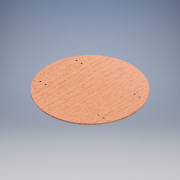
# Autodesk Inventor part: second floor
Saved by Autodesk Inventor 2017 (Build 210142000, 142)
## iProperties
Created: 2019-10-03
Part Number: second floor
Material: Generic
Document SubType Name: Modeling
Designer: User
Density: 1 g/cm^3
Appearance: Weld - Aluminum
Mass: 93.7027 g
Surface Area: 649.465 cm^2
Volume: 93.7027 cm^3
Author: User
Autodesk Inventor part; units mm, degrees
ref_plane "YZ Plane" through (0, 0, 0) normal (1, 0, 0) x (0, 1, 0)
ref_plane "XZ Plane" through (0, 0, 0) normal (0, 1, 0) x (-1, 0, 0)
ref_plane "XY Plane" through (0, 0, 0) normal (0, 0, 1) x (1, 0, 0)
sketch "Sketch1" plane through (0, 0, 0) normal (0, 0, 1) x (1, 0, 0)
  circle A0 centre (0, 0) radius 100
  dimension "d0" = 200
  constraints: 1 centre point, 1 coincident
  measures "d0" diameter of A0
extrude "Extrusion2" add sketch "Sketch1" along normal blind 3
ref_plane "Work Plane1" through (-33, -35, 0) normal (-1, 0, 0) x (0, 0, 1)
sketch "Sketch33" plane through (0, 0, 0) normal (0, 0, -1) x (-1, 0, 0)
  line L0 (-60, 40) -> (-78, 40)
  line L1 (-78, 40) -> (-78, 46)
  line L2 (-78, 46) -> (-60, 46)
  line L3 (-60, 46) -> (-60, 40)
  point P0 (0, 0)
  dimension "d123" = 18
  dimension "d124" = 6
  constraints: 8 end point, 2 parallel, 1 horizontal, 1 perpendicular
  measures "d123" distance of L1.end L2.end
  measures "d124" distance of L0.end L1.end
extrude "Extrusion32" cut sketch "Sketch33" against normal blind 1
mirror "Mirror21" about plane through (0, 0, 0) normal (1, 0, 0) of "Extrusion32"
mirror "Mirror22" about plane through (0, 0, 0) normal (0, 1, 0) of "Extrusion32", "Mirror21"
sketch "Sketch34" plane through (0, 0, 1) normal (0, 0, -1) x (-1, 0, 0)
  circle A0 centre (-75, 43) radius 1.5
  circle A1 centre (-63, 43) radius 1.5
  point P0 (0, 0)
  dimension "d127" = 3
  dimension "d128" = 3
  constraints: 2 centre point
  measures "d127" diameter of A0
  measures "d128" diameter of A1
extrude "Extrusion33" cut sketch "Sketch34" against normal up to next
mirror "Mirror23" about plane through (0, 0, 0) normal (1, 0, 0) of "Extrusion33"
mirror "Mirror24" about plane through (0, 0, 0) normal (0, 1, 0) of "Extrusion33", "Mirror23"
body "Solid2"
